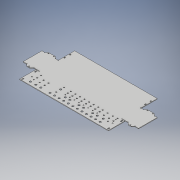
# Autodesk Inventor part: mainCaseFlat
Saved by Autodesk Inventor 2018 (Build 220112000, 112)
## iProperties
Created: 2017-02-09
Part Number: mainCaseFlat
Material: Generic
Document SubType Name: Sheet Metal
Designer: lenord
Density: 1 g/cm^3
Sheet Metal Rule: Default
Appearance: Default
Author: lenord
Autodesk Inventor part; units mm, degrees
ref_plane "YZ Plane" through (0, 0, 0) normal (1, 0, 0) x (0, 1, 0)
ref_plane "XZ Plane" through (0, 0, 0) normal (0, 1, 0) x (-1, 0, 0)
ref_plane "XY Plane" through (0, 0, 0) normal (0, 0, 1) x (1, 0, 0)
sketch "Sketch1" plane through (0, 0, 0) normal (0, 1, 0) x (-1, 0, 0)
  line L0 (257.2308, 49.5858) -> (266.065, 58.42)
  line L1 (266.065, 58.42) -> (283.845, 58.42)
  line L2 (283.845, 58.42) -> (292.6792, 49.5858)
  line L3 (0, 0) -> (0, 139.7) construction
  line L4 (224.155, -55.84) -> (224.155, -142.24)
  line L5 (241.3, 48.26) -> (254.03, 48.26)
  line L6 (295.88, 48.26) -> (313.055, 48.26)
  line L7 (224.155, -53.34) -> (224.155, 139.7) construction
  line L8 (313.055, -53.34) -> (313.055, 48.26)
  line L9 (0, -142.24) -> (0, 139.7) construction
  line L10 (241.3, 48.26) -> (224.155, 48.26)
  line L11 (224.155, 50.8) -> (241.3, 50.8)
  line L12 (241.3, 50.8) -> (241.3, 139.7)
  circle A0 centre (274.955, 54.0029) radius 2.5
  circle A1 centre (253.7883, -59.0829) radius 2.5
  circle A2 centre (283.4217, -59.0829) radius 2.5
  line L13 (274.955, 58.42) -> (274.955, 48.26) construction
  line L14 (226.655, -53.34) -> (237.28, -53.34)
  line L15 (240.4808, -54.6658) -> (249.315, -63.5)
  line L16 (249.315, -63.5) -> (287.895, -63.5)
  line L17 (287.895, -63.5) -> (296.7292, -54.6658)
  line L18 (299.93, -53.34) -> (313.055, -53.34)
  line L19 (241.3, 139.7) -> (0, 139.7)
  line L20 (224.155, -142.24) -> (0, -142.24)
  line L21 (224.155, 50.8) -> (0, 50.8) construction
  line L22 (224.155, 95.25) -> (241.3, 95.25) construction
  line L23 (232.7275, 139.7) -> (232.7275, 50.8) construction
  arc A3 (226.655, -53.34) -> (224.155, -55.84) centre (224.155, -53.34) ccw
  circle A4 centre (218.821, 95.25) radius 2.5
  arc A5 (240.4808, -54.6658) -> (237.28, -53.34) centre (239.155, -53.34) ccw
  arc A6 (299.93, -53.34) -> (296.7292, -54.6658) centre (298.055, -53.34) ccw
  arc A7 (254.03, 48.26) -> (257.2308, 49.5858) centre (255.905, 48.26) ccw
  arc A8 (292.6792, 49.5858) -> (295.88, 48.26) centre (294.005, 48.26) ccw
  line L24 (-257.2308, 49.5858) -> (-266.065, 58.42)
  line L25 (-266.065, 58.42) -> (-283.845, 58.42)
  line L26 (-283.845, 58.42) -> (-292.6792, 49.5858)
  line L27 (-224.155, -55.84) -> (-224.155, -142.24)
  line L28 (-241.3, 48.26) -> (-254.03, 48.26)
  line L29 (-295.88, 48.26) -> (-313.055, 48.26)
  line L30 (-224.155, -53.34) -> (-224.155, 139.7) construction
  line L31 (-313.055, -53.34) -> (-313.055, 48.26)
  line L32 (-241.3, 48.26) -> (-224.155, 48.26)
  line L33 (-224.155, 50.8) -> (-241.3, 50.8)
  line L34 (-241.3, 50.8) -> (-241.3, 139.7)
  circle A9 centre (-274.955, 54.0029) radius 2.5
  circle A10 centre (-253.7883, -59.0829) radius 2.5
  circle A11 centre (-283.4217, -59.0829) radius 2.5
  line L35 (-274.955, 58.42) -> (-274.955, 48.26) construction
  line L36 (-226.655, -53.34) -> (-237.28, -53.34)
  line L37 (-240.4808, -54.6658) -> (-249.315, -63.5)
  line L38 (-249.315, -63.5) -> (-287.895, -63.5)
  line L39 (-287.895, -63.5) -> (-296.7292, -54.6658)
  line L40 (-299.93, -53.34) -> (-313.055, -53.34)
  line L41 (-241.3, 139.7) -> (0, 139.7)
  line L42 (-224.155, -142.24) -> (0, -142.24)
  line L43 (-224.155, 50.8) -> (0, 50.8) construction
  line L44 (-224.155, 95.25) -> (-241.3, 95.25) construction
  line L45 (-232.7275, 139.7) -> (-232.7275, 50.8) construction
  arc A12 (-224.155, -55.84) -> (-226.655, -53.34) centre (-224.155, -53.34) ccw
  circle A13 centre (-218.821, 95.25) radius 2.5
  arc A14 (-237.28, -53.34) -> (-240.4808, -54.6658) centre (-239.155, -53.34) ccw
  arc A15 (-296.7292, -54.6658) -> (-299.93, -53.34) centre (-298.055, -53.34) ccw
  arc A16 (-257.2308, 49.5858) -> (-254.03, 48.26) centre (-255.905, 48.26) ccw
  arc A17 (-295.88, 48.26) -> (-292.6792, 49.5858) centre (-294.005, 48.26) ccw
  circle A18 centre (-198.0051, 229.7957) radius 5
  circle A19 centre (-198.0051, 229.7957) radius 10.75 construction
  line L46 (-206.9953, 246.7597) -> (-189.8978, 246.7597) construction
  line L47 (-189.8978, 246.7597) -> (-189.8978, 242.7114) construction
  line L48 (-189.8978, 242.7114) -> (-206.9953, 242.7114) construction
  line L49 (-206.9953, 242.7114) -> (-206.9953, 246.7597) construction
  circle A20 centre (-179.07, 122.5) radius 5
  circle A21 centre (-179.07, 122.5) radius 10.75 construction
  circle A22 centre (-154.345, 122.5) radius 5
  circle A23 centre (-154.345, 122.5) radius 10.75 construction
  circle A24 centre (-129.62, 122.5) radius 5
  circle A25 centre (-129.62, 122.5) radius 10.75 construction
  circle A26 centre (-104.895, 122.5) radius 5
  circle A27 centre (-104.895, 122.5) radius 10.75 construction
  circle A28 centre (-80.17, 122.5) radius 5
  circle A29 centre (-80.17, 122.5) radius 10.75 construction
  circle A30 centre (-55.445, 122.5) radius 5
  circle A31 centre (-55.445, 122.5) radius 10.75 construction
  circle A32 centre (-30.72, 122.5) radius 5
  circle A33 centre (-30.72, 122.5) radius 10.75 construction
  circle A34 centre (-5.995, 122.5) radius 5
  circle A35 centre (-5.995, 122.5) radius 10.75 construction
  circle A36 centre (18.73, 122.5) radius 5
  circle A37 centre (18.73, 122.5) radius 10.75 construction
  circle A38 centre (43.455, 122.5) radius 5
  circle A39 centre (43.455, 122.5) radius 10.75 construction
  circle A40 centre (68.18, 122.5) radius 5
  circle A41 centre (68.18, 122.5) radius 10.75 construction
  circle A42 centre (92.905, 122.5) radius 5
  circle A43 centre (92.905, 122.5) radius 10.75 construction
  circle A44 centre (-141.9825, 101.4838) radius 5
  circle A45 centre (-141.9825, 101.4838) radius 10.75 construction
  circle A46 centre (-154.9768, 228.869) radius 10.5 construction
  circle A47 centre (-154.9768, 228.869) radius 3.5
  line L50 (-161.7198, 245.7266) -> (-144.4768, 245.7266) construction
  line L51 (-144.4768, 245.7266) -> (-144.4768, 241.5684) construction
  line L52 (-144.4768, 241.5684) -> (-161.7198, 241.5684) construction
  line L53 (-161.7198, 241.5684) -> (-161.7198, 245.7266) construction
  circle A48 centre (-129.62, 75.565) radius 3.5
  circle A49 centre (-129.62, 75.565) radius 10.5 construction
  circle A50 centre (-114.9114, 228.3591) radius 2.5
  line L54 (-118.333, 235.7128) -> (-112.852, 235.7128) construction
  line L55 (-112.852, 235.7128) -> (-112.852, 232.4648) construction
  line L56 (-112.852, 232.4648) -> (-118.333, 232.4648) construction
  line L57 (-118.333, 232.4648) -> (-118.333, 235.7128) construction
  circle A51 centre (-96.09, 228.869) radius 3.25
  circle A52 centre (-96.09, 228.869) radius 6.5 construction
  circle A53 centre (-129.62, 89.215) radius 2.5
  circle A54 centre (-129.62, 59.055) radius 3.25
  circle A55 centre (-129.62, 59.055) radius 6.5 construction
  circle A56 centre (-104.895, 89.215) radius 2.5
  circle A57 centre (-104.895, 75.565) radius 10.5 construction
  circle A58 centre (-104.895, 75.565) radius 3.5
  circle A59 centre (-104.895, 59.055) radius 6.5 construction
  circle A60 centre (-104.895, 59.055) radius 3.25
  circle A61 centre (-80.17, 89.215) radius 2.5
  circle A62 centre (-80.17, 75.565) radius 10.5 construction
  circle A63 centre (-80.17, 75.565) radius 3.5
  circle A64 centre (-80.17, 59.055) radius 6.5 construction
  circle A65 centre (-80.17, 59.055) radius 3.25
  circle A66 centre (-55.445, 89.215) radius 2.5
  circle A67 centre (-55.445, 75.565) radius 10.5 construction
  circle A68 centre (-55.445, 75.565) radius 3.5
  circle A69 centre (-55.445, 59.055) radius 6.5 construction
  circle A70 centre (-55.445, 59.055) radius 3.25
  circle A71 centre (-30.72, 89.215) radius 2.5
  circle A72 centre (-30.72, 75.565) radius 10.5 construction
  circle A73 centre (-30.72, 75.565) radius 3.5
  circle A74 centre (-30.72, 59.055) radius 6.5 construction
  circle A75 centre (-30.72, 59.055) radius 3.25
  circle A76 centre (-5.995, 89.215) radius 2.5
  circle A77 centre (-5.995, 75.565) radius 10.5 construction
  circle A78 centre (-5.995, 75.565) radius 3.5
  circle A79 centre (-5.995, 59.055) radius 6.5 construction
  circle A80 centre (-5.995, 59.055) radius 3.25
  circle A81 centre (18.73, 89.215) radius 2.5
  circle A82 centre (18.73, 75.565) radius 10.5 construction
  circle A83 centre (18.73, 75.565) radius 3.5
  circle A84 centre (18.73, 59.055) radius 6.5 construction
  circle A85 centre (18.73, 59.055) radius 3.25
  circle A86 centre (43.455, 89.215) radius 2.5
  circle A87 centre (43.455, 75.565) radius 10.5 construction
  circle A88 centre (43.455, 75.565) radius 3.5
  circle A89 centre (43.455, 59.055) radius 6.5 construction
  circle A90 centre (43.455, 59.055) radius 3.25
  circle A91 centre (-117.2575, 101.4838) radius 10.75 construction
  circle A92 centre (-117.2575, 101.4838) radius 5
  circle A93 centre (-67.8075, 101.4838) radius 10.75 construction
  circle A94 centre (-67.8075, 101.4838) radius 5
  circle A95 centre (-43.0825, 101.4838) radius 5
  circle A96 centre (-43.0825, 101.4838) radius 10.75 construction
  circle A97 centre (6.3675, 101.4838) radius 10.75 construction
  circle A98 centre (6.3675, 101.4838) radius 5
  circle A99 centre (31.0925, 101.4838) radius 5
  circle A100 centre (31.0925, 101.4838) radius 10.75 construction
  circle A101 centre (-158.0537, 81.7562) radius 3.5
  circle A102 centre (-158.0537, 81.7562) radius 10.5 construction
  circle A103 centre (-158.0537, 61.1188) radius 6.5 construction
  circle A104 centre (-158.0537, 61.1188) radius 3.25
  line L58 (-240.5298, 172.4522) -> (-235.6099, 172.4522) construction
  line L59 (-235.6099, 172.4522) -> (-235.6099, 167.5324) construction
  line L60 (-235.6099, 167.5324) -> (-240.5298, 167.5324) construction
  line L61 (-240.5298, 167.5324) -> (-240.5298, 172.4522) construction
  circle A105 centre (-172.2706, 99.2981) radius 5
  circle A106 centre (-172.2706, 99.2981) radius 10.75 construction
  circle A107 centre (-186.4875, 81.7562) radius 10.5 construction
  circle A108 centre (-186.4875, 81.7562) radius 3.5
  circle A109 centre (-186.4875, 61.1188) radius 6.5 construction
  circle A110 centre (-186.4875, 61.1188) radius 3.25
  circle A111 centre (80.5425, 101.4838) radius 6.5 construction
  circle A112 centre (80.5425, 101.4838) radius 3.25
  circle A113 centre (80.5425, 77.3538) radius 5
  circle A114 centre (80.5425, 77.3538) radius 10.75 construction
  circle A115 centre (80.5425, 59.055) radius 6.5 construction
  circle A116 centre (80.5425, 59.055) radius 3.25
  line L62 (-102.3863, 240.0967) -> (-90.7748, 240.0967) construction
  line L63 (-90.7748, 240.0967) -> (-90.7748, 236.8585) construction
  line L64 (-90.7748, 236.8585) -> (-102.3863, 236.8585) construction
  line L65 (-102.3863, 236.8585) -> (-102.3863, 240.0967) construction
  circle A117 centre (-210.185, 81.7562) radius 3.5
  circle A118 centre (-210.185, 81.7562) radius 10.5 construction
  circle A119 centre (-210.185, 59.055) radius 6.5 construction
  circle A120 centre (-210.185, 59.055) radius 3.25
  circle A121 centre (-210.185, 68.58) radius 2.5
  line L66 (-330.0315, 119.0778) -> (-248.3728, 119.0778) construction
  line L67 (-248.3728, 119.0778) -> (-248.3728, 119.8138) construction
  line L68 (-248.3728, 119.8138) -> (-330.0315, 119.8138) construction
  line L69 (-330.0315, 119.8138) -> (-330.0315, 119.0778) construction
  line L70 (59.1952, 159.9316) -> (63.2213, 159.9316) construction
  line L71 (63.2213, 159.9316) -> (63.2213, 155.9055) construction
  line L72 (63.2213, 155.9055) -> (59.1952, 155.9055) construction
  line L73 (59.1952, 155.9055) -> (59.1952, 159.9316) construction
  circle A122 centre (-197.861, 99.2981) radius 3.25
  circle A123 centre (-197.861, 99.2981) radius 6.5 construction
  line L74 (-202.7888, 31.6249) -> (-199.5308, 31.6249) construction
  line L75 (-199.5308, 31.6249) -> (-199.5308, 28.367) construction
  line L76 (-199.5308, 28.367) -> (-202.7888, 28.367) construction
  line L77 (-202.7888, 28.367) -> (-202.7888, 31.6249) construction
  circle A124 centre (199.39, 122.5) radius 10.75 construction
  circle A125 centre (199.39, 122.5) radius 5
  circle A126 centre (199.39, 85.95) radius 3.5
  circle A127 centre (199.39, 85.95) radius 10.5 construction
  circle A128 centre (199.39, 104.225) radius 2.5
  circle A129 centre (199.39, 64.95) radius 3.25
  circle A130 centre (199.39, 64.95) radius 6.5 construction
  circle A131 centre (170.053, 122.5) radius 5
  circle A132 centre (170.053, 122.5) radius 10.75 construction
  line L78 (193.0383, 161.4795) -> (214.3619, 161.4795) construction
  line L79 (214.3619, 161.4795) -> (214.3619, 143.1563) construction
  line L80 (214.3619, 143.1563) -> (193.0383, 143.1563) construction
  line L81 (193.0383, 143.1563) -> (193.0383, 161.4795) construction
  line L82 (164.7951, 158.772) -> (183.7945, 158.772) construction
  line L83 (183.7945, 158.772) -> (183.7945, 139.7726) construction
  line L84 (183.7945, 139.7726) -> (164.7951, 139.7726) construction
  line L85 (164.7951, 139.7726) -> (164.7951, 158.772) construction
  circle A133 centre (170.053, 101.4838) radius 6.5 construction
  circle A134 centre (170.053, 101.4838) radius 3.25
  circle A135 centre (170.053, 80.4838) radius 3.5
  circle A136 centre (170.053, 80.4838) radius 10.5 construction
  line L86 (134.8346, 158.5069) -> (158.6119, 158.5069) construction
  line L87 (158.6119, 158.5069) -> (158.6119, 140.3043) construction
  line L88 (158.6119, 140.3043) -> (134.8346, 140.3043) construction
  line L89 (134.8346, 140.3043) -> (134.8346, 158.5069) construction
  circle A137 centre (143.178, 122.5) radius 10.75 construction
  circle A138 centre (143.178, 122.5) radius 5
  circle A139 centre (143.178, 101.4838) radius 3.25
  circle A140 centre (143.178, 101.4838) radius 6.5 construction
  circle A141 centre (143.178, 80.4838) radius 10.5 construction
  circle A142 centre (143.178, 80.4838) radius 3.5
  line L90 (239.155, -53.34) -> (240.4808, -54.6658) construction
  line L91 (298.055, -53.34) -> (296.7292, -54.6658) construction
  line L92 (244.8979, -59.0829) -> (292.3121, -59.0829) construction
  line L93 (-296.7292, -54.6658) -> (-298.055, -53.34) construction
  line L94 (-240.4808, -54.6658) -> (-239.155, -53.34) construction
  line L95 (-292.3121, -59.0829) -> (-244.8979, -59.0829) construction
  line L96 (-294.005, 48.26) -> (-292.735, 49.53) construction
  line L97 (-255.905, 48.26) -> (-257.175, 49.53) construction
  arc A143 (224.155, 50.8) -> (224.155, 48.26) centre (224.155, 49.53) ccw
  line L98 (255.905, 48.26) -> (257.2308, 49.5858) construction
  line L99 (292.6792, 49.5858) -> (294.005, 48.26) construction
  line L100 (261.6479, 54.0029) -> (288.2621, 54.0029) construction
  line L101 (-224.155, 48.26) -> (-224.155, 50.8) construction
  arc A144 (-224.155, 48.26) -> (-224.155, 50.8) centre (-224.155, 49.53) ccw
  line L102 (-288.2621, 54.0029) -> (-261.6479, 54.0029) construction
  line L103 (232.7275, 136.0932) -> (232.7275, 136.0932)
  line L104 (235.4707, 133.35) -> (235.4707, 127.0406)
  line L105 (232.7275, 124.2974) -> (232.7275, 124.2974)
  line L106 (229.9843, 127.0406) -> (229.9843, 133.35)
  arc A145 (232.7275, 136.0932) -> (229.9843, 133.35) centre (232.7275, 133.35) ccw
  arc A146 (235.4707, 133.35) -> (232.7275, 136.0932) centre (232.7275, 133.35) ccw
  arc A147 (229.9843, 127.0406) -> (232.7275, 124.2974) centre (232.7275, 127.0406) ccw
  arc A148 (232.7275, 124.2974) -> (235.4707, 127.0406) centre (232.7275, 127.0406) ccw
  line L107 (232.7275, 66.2026) -> (232.7275, 66.2026)
  line L108 (235.4707, 63.4594) -> (235.4707, 57.15)
  line L109 (232.7275, 54.4068) -> (232.7275, 54.4068)
  line L110 (229.9843, 57.15) -> (229.9843, 63.4594)
  arc A149 (229.9843, 57.15) -> (232.7275, 54.4068) centre (232.7275, 57.15) ccw
  arc A150 (232.7275, 54.4068) -> (235.4707, 57.15) centre (232.7275, 57.15) ccw
  arc A151 (235.4707, 63.4594) -> (232.7275, 66.2026) centre (232.7275, 63.4594) ccw
  arc A152 (232.7275, 66.2026) -> (229.9843, 63.4594) centre (232.7275, 63.4594) ccw
  line L111 (218.821, -79.2233) -> (218.821, -79.2233)
  line L112 (221.321, -81.7233) -> (221.321, -84.2233)
  line L113 (218.821, -86.7233) -> (218.821, -86.7233)
  line L114 (216.321, -84.2233) -> (216.321, -81.7233)
  arc A153 (218.821, -79.2233) -> (216.321, -81.7233) centre (218.821, -81.7233) ccw
  arc A154 (221.321, -81.7233) -> (218.821, -79.2233) centre (218.821, -81.7233) ccw
  arc A155 (216.321, -84.2233) -> (218.821, -86.7233) centre (218.821, -84.2233) ccw
  arc A156 (218.821, -86.7233) -> (221.321, -84.2233) centre (218.821, -84.2233) ccw
  line L115 (221.321, -82.9733) -> (216.321, -82.9733) construction
  line L116 (218.821, -108.8567) -> (218.821, -108.8567)
  line L117 (221.321, -111.3567) -> (221.321, -113.8567)
  line L118 (218.821, -116.3567) -> (218.821, -116.3567)
  line L119 (216.321, -113.8567) -> (216.321, -111.3567)
  arc A157 (218.821, -108.8567) -> (216.321, -111.3567) centre (218.821, -111.3567) ccw
  arc A158 (221.321, -111.3567) -> (218.821, -108.8567) centre (218.821, -111.3567) ccw
  arc A159 (218.821, -116.3567) -> (221.321, -113.8567) centre (218.821, -113.8567) ccw
  arc A160 (216.321, -113.8567) -> (218.821, -116.3567) centre (218.821, -113.8567) ccw
  line L120 (216.321, -112.6067) -> (221.321, -112.6067) construction
  line L121 (-232.7275, 136.0932) -> (-232.7275, 136.0932)
  line L122 (-235.4707, 133.35) -> (-235.4707, 127.0406)
  line L123 (-232.7275, 124.2974) -> (-232.7275, 124.2974)
  line L124 (-229.9843, 127.0406) -> (-229.9843, 133.35)
  arc A161 (-229.9843, 133.35) -> (-232.7275, 136.0932) centre (-232.7275, 133.35) ccw
  arc A162 (-232.7275, 136.0932) -> (-235.4707, 133.35) centre (-232.7275, 133.35) ccw
  arc A163 (-232.7275, 124.2974) -> (-229.9843, 127.0406) centre (-232.7275, 127.0406) ccw
  arc A164 (-235.4707, 127.0406) -> (-232.7275, 124.2974) centre (-232.7275, 127.0406) ccw
  line L125 (-232.7275, 66.2026) -> (-232.7275, 66.2026)
  line L126 (-235.4707, 63.4594) -> (-235.4707, 57.15)
  line L127 (-232.7275, 54.4068) -> (-232.7275, 54.4068)
  line L128 (-229.9843, 57.15) -> (-229.9843, 63.4594)
  arc A165 (-232.7275, 54.4068) -> (-229.9843, 57.15) centre (-232.7275, 57.15) ccw
  arc A166 (-235.4707, 57.15) -> (-232.7275, 54.4068) centre (-232.7275, 57.15) ccw
  arc A167 (-232.7275, 66.2026) -> (-235.4707, 63.4594) centre (-232.7275, 63.4594) ccw
  arc A168 (-229.9843, 63.4594) -> (-232.7275, 66.2026) centre (-232.7275, 63.4594) ccw
  line L129 (-218.821, -79.2233) -> (-218.821, -79.2233)
  line L130 (-221.321, -81.7233) -> (-221.321, -84.2233)
  line L131 (-218.821, -86.7233) -> (-218.821, -86.7233)
  line L132 (-216.321, -84.2233) -> (-216.321, -81.7233)
  arc A169 (-216.321, -81.7233) -> (-218.821, -79.2233) centre (-218.821, -81.7233) ccw
  arc A170 (-218.821, -79.2233) -> (-221.321, -81.7233) centre (-218.821, -81.7233) ccw
  arc A171 (-218.821, -86.7233) -> (-216.321, -84.2233) centre (-218.821, -84.2233) ccw
  arc A172 (-221.321, -84.2233) -> (-218.821, -86.7233) centre (-218.821, -84.2233) ccw
  line L133 (-221.321, -82.9733) -> (-216.321, -82.9733) construction
  line L134 (-218.821, -108.8567) -> (-218.821, -108.8567)
  line L135 (-221.321, -111.3567) -> (-221.321, -113.8567)
  line L136 (-218.821, -116.3567) -> (-218.821, -116.3567)
  line L137 (-216.321, -113.8567) -> (-216.321, -111.3567)
  arc A173 (-216.321, -111.3567) -> (-218.821, -108.8567) centre (-218.821, -111.3567) ccw
  arc A174 (-218.821, -108.8567) -> (-221.321, -111.3567) centre (-218.821, -111.3567) ccw
  arc A175 (-221.321, -113.8567) -> (-218.821, -116.3567) centre (-218.821, -113.8567) ccw
  arc A176 (-218.821, -116.3567) -> (-216.321, -113.8567) centre (-218.821, -113.8567) ccw
  line L138 (-216.321, -112.6067) -> (-221.321, -112.6067) construction
  point P0 (232.7275, 95.25)
  point P1 (-232.7275, 95.25)
  dimension "d37" = 224.155
  dimension "d38" = 10.16
  dimension "d39" = 19.05
  dimension "d45" = 45
  dimension "d64" = 2.54
  dimension "d66" = 5
  dimension "d69" = 15
  dimension "d70" = 101.6
  dimension "d71" = 88.9
  dimension "d74" = 241.3
  dimension "d77" = 139.7
  dimension "d81" = 5.334
  dimension "d83" = 29.6333
  dimension "d84" = 59.2667
  dimension "d87" = 3.75
  dimension "d88" = 10
  dimension "d89" = 21.5
  dimension "d90" = 62.23
  dimension "d91" = 17.2
  dimension "d94" = 24.725
  dimension "d99" = 99.3175
  dimension "d100" = 21.0162
  dimension "d109" = 21
  dimension "d110" = 7
  dimension "d111" = 5
  dimension "d112" = 13
  dimension "d113" = 6.5
  dimension "d114" = 8.255
  dimension "d115" = 16.51
  dimension "d116" = 13.65
  dimension "d117" = 111.68
  dimension "d120" = 24.725
  dimension "d127" = 24.725
  dimension "d134" = 74.175
  dimension "d139" = 10.3187
  dimension "d140" = 20.6375
  dimension "d141" = 83.2463
  dimension "d144" = 28.4337
  dimension "d149" = 69.0294
  dimension "d150" = 17.5419
  dimension "d151" = 321.8425
  dimension "d152" = 24.13
  dimension "d153" = 9.525
  dimension "d154" = 31.115
  dimension "d155" = 43.439
  dimension "d156" = 18.275
  dimension "d157" = 18.275
  dimension "d158" = 21
  dimension "d159" = 41.91
  dimension "d160" = 17.2
  dimension "d161" = 21
  dimension "d162" = 26.875
  dimension "d163" = 71.247
  dimension "d164" = 88.9
  dimension "d166" = 88.9
  dimension "d169" = 10.16
  dimension "d171" = 135
  dimension "d172" = 135
  dimension "d173" = 15
  dimension "d174" = 29.6333
  dimension "d175" = 59.2667
  dimension "d176" = 135
  dimension "d177" = 31.75
  dimension "d178" = 135
  constraints: 190 end point, 177 centre point, 88 point on circle, 83 symmetric about line, 69 equal radius, 68 coincident, 34 tangent, 23 midpoint, 22 point on line, 18 horizontal, 15 collinear, 15 vertical alignment, 14 horizontal alignment, 13 equal length, 10 perpendicular, 9 parallel, 3 vertical, 186 other
  measures "d37" distance from line of L4 L3.start
  measures "d38" distance between parallel lines of L6 L1
  measures "d39" distance of point (294.005, 48.26) L6.end
  measures "d45" angle of L2 L6
  measures "d64" distance between parallel lines of L10 L11
  measures "d66" diameter of A0
  measures "d69" distance of point (298.055, -53.34) L8.start
  measures "d70" distance between parallel lines of L6 L18
  measures "d71" distance of L11.end L12.end
  measures "d74" distance between parallel lines of L12 L3
  measures "d77" distance from line of L3.start L19
  measures "d81" distance from line of L7 A4.centre
  measures "d83" distance from line of A2.centre L8
  measures "d84" distance from line of L8 A1.centre
  measures "d87" diameter of A5
  measures "d88" diameter of A18
  measures "d89" diameter of A19
  measures "d90" distance from line of A20.centre L34
  measures "d91" distance from line of L41 A20.centre
  measures "d94" distance of A20.centre A22.centre
  measures "d99" distance from line of A44.centre L34
  measures "d100" vertical distance of A44.centre A30.centre
  measures "d109" diameter of A46
  measures "d110" diameter of A47
  measures "d111" diameter of A50
  measures "d112" diameter of A52
  measures "d113" diameter of A51
  measures "d114" distance from line of A54.centre L43
  measures "d115" distance of A49.centre A54.centre
  measures "d116" distance of A49.centre A53.centre
  measures "d117" distance from line of A48.centre L34
  measures "d120" distance of A53.centre A56.centre
  measures "d127" distance of A45.centre A91.centre
  measures "d134" distance of A45.centre A93.centre
  measures "d139" distance from line of A103.centre L43
  measures "d140" distance of A101.centre A104.centre
  measures "d141" distance from line of A101.centre L34
  measures "d144" distance of A102.centre A107.centre
  measures "d149" distance from line of A105.centre L34
  measures "d150" vertical distance of A105.centre A107.centre
  measures "d151" distance from line of A111.centre L34
  measures "d152" distance of A113.centre A112.centre
  measures "d153" distance of A121.centre A120.centre
  measures "d154" distance from line of A120.centre L34
  measures "d155" distance from line of A122.centre L34
  measures "d156" distance of A124.centre A128.centre
  measures "d157" distance of A128.centre A126.centre
  measures "d158" distance of A126.centre A129.centre
  measures "d159" distance from line of A124.centre L12
  measures "d160" distance from line of L19 A124.centre
  measures "d161" distance of A135.centre A133.centre
  measures "d162" distance of A132.centre A137.centre
  measures "d163" distance from line of L12 A132.centre
  measures "d164" distance between parallel lines of L14 L20
  measures "d166" distance from line of L8 L7.start
  measures "d169" distance from line of point (298.055, -53.34) L16
  measures "d171" angle of L18 L91
  measures "d172" angle of L90 L14
  measures "d173" distance from line of point (239.155, -53.34) L4
  measures "d174" distance from line of A11.centre L31
  measures "d175" distance from line of A10.centre L31
  measures "d176" angle of L26 L29
  measures "d177" horizontal distance of L98.start A143.centre
  measures "d178" angle of L0 L5
extrude "Plate2" add sketch "Sketch1" along normal blind 3.048 contours L0 L1 L2 A8 L6 L8 L18 A6 L17 L16 L15 A5 L14 A3 L4 L20 L42 L27 A12 L36 A14 L37 L38 L39 A15 L40 L31 L29 A17 L26 L25 L24 A16 L28 L32 A144 L33 L34 L41 L19 L12 L11 A143 L10 L5 A7
equation "\"d37\" = 0.5 * d36"
equation "\"BendRadius\" = Thickness"
equation "\"BendReliefWidth\" = Thickness"
equation "\"BendReliefDepth\" = 0.5 * Thickness"
equation "\"CornerReliefSize\" = 4 * Thickness"
equation "\"MinimumRemnant\" = 2 * Thickness"
equation "\"TransitionRadius\" = BendRadius"
equation "\"JacobiRadiusSize\" = Thickness"
equation "\"GapSize\" = Thickness"
equation "\"d14\" = BendRadius"
equation "\"d56\" = d55"
equation "\"d36\" = 448.31"
equation "\"Thickness\" = 3.048"
equation "\"d55\" = 88.9"
body "Solid2"
